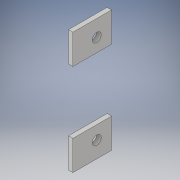
# Autodesk Inventor part: Fixador traseiro
Saved by Autodesk Inventor 2019 (Build 230136000, 136)
## iProperties
Created: 2021-05-28
Part Number: Fixador traseiro
Material: Generic
Document SubType Name: Modeling
Designer: hoope
Density: 1 g/cm^3
Appearance: Default
Author: hoope
Autodesk Inventor part; units mm, degrees
ref_plane "YZ Plane" through (0, 0, 0) normal (1, 0, 0) x (0, 1, 0)
ref_plane "XZ Plane" through (0, 0, 0) normal (0, 1, 0) x (-1, 0, 0)
ref_plane "XY Plane" through (0, 0, 0) normal (0, 0, 1) x (1, 0, 0)
sketch "Esboço1" plane through (0, 0, 0) normal (0, 1, 0) x (-1, 0, 0)
  line L0 (0, 0.1088) -> (3, 0.1088)
  line L1 (3, 0.1088) -> (3, -25.8912)
  line L2 (3, -25.8912) -> (0, -25.8912)
  line L3 (0, -25.8912) -> (0, 0.1088)
  point P0 (0, 0)
  dimension "d0" = 3
  dimension "d1" = 26
  constraints: 8 end point, 2 parallel, 1 horizontal, 1 perpendicular
  measures "d0" distance of L1.end L2.end
  measures "d1" distance of L0.end L1.end
extrude "Extrusão1" add sketch "Esboço1" along normal blind 82
sketch "Esboço2" plane through (0, 0, 0.1088) normal (1, 0, 0) x (0, 0, -1)
  line L0 (26, 0) -> (26, 82) projected
  line L1 (0, 0) -> (0, 82) projected
  line L2 (26, 20) -> (0, 20)
  line L3 (0, 20) -> (0, 62)
  line L4 (0, 62) -> (26, 62)
  line L5 (26, 62) -> (26, 20)
  line L6 (0, 82) -> (26, 82) projected
  point P0 (0.1088, 0)
  dimension "d4" = 42
  dimension "d5" = 20
  constraints: 8 end point, 2 parallel, 2 point on line, 1 horizontal, 1 perpendicular
  measures "d4" distance of L2.end L3.end
  measures "d5" distance between parallel lines of L6 L4
extrude "Extrusão2" cut sketch "Esboço2" against normal blind 42 contours L2 L1 L4 L0
sketch "Esboço3" plane through (0, 82, 0.1088) normal (1, 0, 0) x (0, 0, -1)
  circle A0 centre (16, -11) radius 3
  circle A1 centre (16, -71) radius 3
  line L0 (0, -20) -> (26, -20) projected
  line L1 (26, -62) -> (0, -62) projected
  line L2 (26, -20) -> (26, 0) projected
  line L3 (26, -82) -> (26, -62) projected
  point P0 (0.1088, -82)
  dimension "d8" = 6
  dimension "d9" = 6
  dimension "d10" = 9
  dimension "d11" = 9
  dimension "d12" = 10
  dimension "d13" = 10
  constraints: 2 centre point
  measures "d8" diameter of A0
  measures "d9" diameter of A1
  measures "d10" distance from line of L0 A0.centre
  measures "d11" distance from line of L1 A1.centre
  measures "d12" distance from line of L2 A0.centre
  measures "d13" distance from line of L3 A1.centre
extrude "Extrusão3" cut sketch "Esboço3" against normal blind 42
